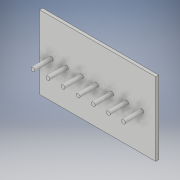
# Autodesk Inventor part: gearbasephonecase
Saved by Autodesk Inventor 2018 (Build 220112000, 112)
## iProperties
Created: 2019-03-18
Part Number: gearbasephonecase
Material: Generic
Document SubType Name: Modeling
Designer: F8PLTW
Density: 1 g/cm^3
Appearance: Default
Author: F8PLTW
Autodesk Inventor part; units mm, degrees
ref_plane "YZ Plane" through (0, 0, 0) normal (1, 0, 0) x (0, 1, 0)
ref_plane "XZ Plane" through (0, 0, 0) normal (0, 1, 0) x (-1, 0, 0)
ref_plane "XY Plane" through (0, 0, 0) normal (0, 0, 1) x (1, 0, 0)
sketch "Sketch1" plane through (0, 0, 0) normal (0, 0, 1) x (1, 0, 0)
  line L0 (-22.1112, 10.3171) -> (130.2888, 10.3171)
  line L1 (130.2888, 10.3171) -> (130.2888, -65.8829)
  line L2 (130.2888, -65.8829) -> (-22.1112, -65.8829)
  line L3 (-22.1112, -65.8829) -> (-22.1112, 10.3171)
  point P0 (0, 0)
  dimension "d0" = 152.4
  dimension "d1" = 76.2
  constraints: 8 end point, 2 parallel, 1 horizontal, 1 perpendicular
  measures "d0" distance of L1.end L2.end
  measures "d1" distance of L0.end L1.end
extrude "Extrusion1" add sketch "Sketch1" along normal blind 3.175
sketch "Sketch2" plane through (0, 0, 3.175) normal (0, 0, 1) x (1, 0, 0)
  circle A0 centre (-10.0607, -27.9271) radius 2
  circle A1 centre (5.6233, -27.9271) radius 2
  circle A2 centre (21.3073, -27.9271) radius 2
  circle A3 centre (36.9913, -27.9271) radius 2
  circle A4 centre (52.6753, -27.9271) radius 2
  circle A5 centre (68.3593, -27.9271) radius 2
  circle A6 centre (84.0433, -27.9271) radius 2
  point P0 (0, 0)
  dimension "d4" = 4
  dimension "d5" = 4
  dimension "d6" = 4
  dimension "d7" = 11.684
  dimension "d8" = 11.684
  dimension "d9" = 4
  dimension "d10" = 11.684
  dimension "d11" = 4
  dimension "d12" = 4
  dimension "d13" = 4
  dimension "d14" = 11.684
  dimension "d15" = 11.684
  dimension "d16" = 11.684
  constraints: 7 centre point
  measures "d4" diameter of A0
  measures "d5" diameter of A1
  measures "d6" diameter of A2
  measures "d9" diameter of A3
  measures "d11" diameter of A4
  measures "d12" diameter of A5
  measures "d13" diameter of A6
extrude "Extrusion2" add sketch "Sketch2" along normal blind 19.05
sketch "Sketch3" plane through (130.2888, -65.8829, 0) normal (1, 0, 0) x (0, 0, -1)
  line L0 (-11.1509, 83.1688) -> (7.2167, 83.1688)
  line L1 (7.2167, 83.1688) -> (7.2167, -5.5026)
  line L2 (7.2167, -5.5026) -> (-11.1509, -5.5026)
  line L3 (-11.1509, -5.5026) -> (-11.1509, 83.1688)
  point P0 (0, 65.8829)
  constraints: 8 end point, 2 parallel, 1 horizontal, 1 perpendicular
extrude "Extrusion3" cut sketch "Sketch3" against normal blind 31.75
body "Solid1"
